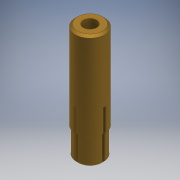
# Autodesk Inventor part: Pino_contato_L
Saved by Autodesk Inventor 2018 (Build 220112000, 112)
## iProperties
Created: 2021-03-23
Part Number: Pino_contato_L
Material: Genérico
Document SubType Name: Modeling
Designer: nilton
Density: 1 g/cm^3
Appearance: Latão - Acetinado
Author: nilton
Autodesk Inventor part; units mm, degrees
note: some values were not read from the file. Chosen so that the rebuilt part matches the saved one: direction of "Furo3".
ref_plane "YZ Plane" through (0, 0, 0) normal (1, 0, 0) x (0, 1, 0)
ref_plane "XY Plane" through (0, 0, 0) normal (0, 0, 1) x (1, 0, 0)
sketch "Esboço1" plane through (0, 0, 0) normal (0, 0, 1) x (1, 0, 0)
  circle A0 centre (0, 0) radius 3.5
  dimension "d0" = 7
  constraints: 1 centre point, 1 coincident
  measures "d0" diameter of A0
extrude "Extrusão1" add sketch "Esboço1" along normal mid plane 27.5
sketch "Esboço2" plane through (0, 0, 13.75) normal (0, 0, 1) x (1, 0, 0)
  point P0 (0, 0)
  point P1 (0, 0)
  constraints: 1 coincident
hole "Furo1" at (0, 0, 13.75) direction (0, 0, -1) diameter 3.2 depth 7 tip angle 118
sketch "Esboço3" plane through (0, 0, -13.75) normal (0, 0, -1) x (-1, 0, 0)
  point P0 (0, 0)
  point P1 (0, 0)
  constraints: 1 coincident
hole "Furo2" at (0, 0, -13.75) direction (0, 0, 1) diameter 4.5 depth 18 tip angle 118
sketch "Esboço4" plane through (0, 0, -13.75) normal (0, 0, -1) x (-1, 0, 0)
  circle A0 centre (0, 0) radius 3.5 projected
  circle A1 centre (0, 0) radius 3.25
  dimension "d18" = 6.5
  constraints: 1 centre point, 1 coincident
  measures "d18" diameter of A1
extrude "Extrusão2" cut sketch "Esboço4" against normal blind 6.5
sketch "Esboço5" plane through (0, 0, 0) normal (1, 0, 0) x (0, 1, 0)
  line L0 (3.5, -7.25) -> (3.5, 13.75) projected
  line L1 (3.5, -1.75) -> (-3.5, -1.75)
  line L2 (-3.5, -1.75) -> (-3.5, -13.75)
  line L3 (3.5, -13.75) -> (3.5, -1.75)
  line L4 (-3.5, -7.25) -> (-3.5, 13.75) projected
  line L5 (-3.25, -13.75) -> (3.25, -13.75) projected
  line L6 (3.25, -13.75) -> (3.25, -7.25) projected
  line L7 (3.5, -13.75) -> (-3.5, -13.75)
  point P0 (0, 0)
  dimension "d23" = 12
  constraints: 8 end point, 2 collinear, 2 horizontal, 1 parallel, 1 perpendicular, 1 point on line
  measures "d23" distance of L3.start L1.start
extrude "Extrusão3" cut sketch "Esboço5" along normal mid plane 0.5
sketch "Esboço6" plane through (0, 0, 0) normal (0, 1, 0) x (-1, 0, 0)
  line L0 (-3.5, -7.25) -> (-3.5, 13.75) projected
  line L1 (3.5, -7.25) -> (3.5, 13.75) projected
  line L2 (-0.25, -1.75) -> (0.25, -1.75) projected
  line L3 (-3.5, -13.75) -> (3.5, -13.75)
  line L4 (3.5, -13.75) -> (3.5, -1.75)
  line L5 (3.5, -1.75) -> (-3.5, -1.75)
  line L6 (-3.5, -1.75) -> (-3.5, -13.75)
  line L7 (-3.25, -13.75) -> (-0.25, -13.75) projected
  line L8 (0.25, -13.75) -> (3.25, -13.75) projected
  point P0 (0, 0)
  constraints: 8 end point, 3 collinear, 2 parallel, 1 horizontal, 1 perpendicular, 1 point on line
extrude "Extrusão4" cut sketch "Esboço6" along normal mid plane 0.5
ref_plane "Plano de trabalho1" through (0, 3.5, 0) normal (0, 1, 0) x (-1, 0, 0)
sketch "Esboço7" plane through (0, 3.5, 0) normal (0, 1, 0) x (-1, 0, 0)
  line L0 (-1.6, 13.75) -> (1.6, 13.75) projected
  line L1 (0, 13.75) -> (0, 10.75) construction
  point P0 (0, 0)
  dimension "d28" = 3
  constraints: 2 end point, 1 midpoint, 1 vertical
  measures "d28" distance of L1.start L1.end
hole "Furo3" at (0, 3.5, 10.75) direction (0, -1, 0) diameter 2.459 end up to surface thread size "M3x0.5" class "6H" standard "ANSI Metric M Profile"
chamfer "Chanfro1" distance 0.5 angle 45 5 edges at (-3.5, 0, 13.75) (-2.2981, 2.2981, -13.75) (-2.2981, -2.2981, -13.75) (2.2981, -2.2981, -13.75) (2.2981, 2.2981, -13.75)
